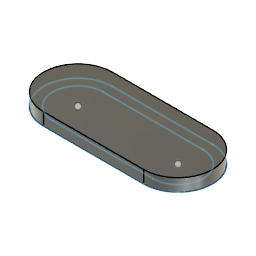
CNC (Autodesk Fusion 360 design; units mm, degrees)
part number: 2025-10-28-20-52-08-507
Autodesk Fusion 360 part; units mm, degrees
sketch "Sketch1" plane through (0, 0, 0) normal (0, 0, 1) x (1, 0, 0)
  line L0 (0.0245, 49.9718) -> (160.0245, 49.9718)
  line L1 (0.0257, -60.0282) -> (160.0257, -60.0282)
  arc A0 (0.0245, 49.9718) -> (0.0257, -60.0282) centre (-0.0009, -5.0282) ccw
  arc A1 (160.0257, -60.0282) -> (160.0245, 49.9718) centre (160.0195, -5.0282) ccw
  line L2 (80.0245, 49.9718) -> (80.0245, 34.9718) construction
  line L3 (0.0245, 34.9718) -> (160.0245, 34.9718)
  line L4 (80.0257, -60.0282) -> (80.0257, -45.0282) construction
  line L5 (0.0257, -45.0282) -> (160.0257, -45.0282)
  line L6 (160.0245, 49.9718) -> (160.0245, 34.9718) construction
  line L7 (160.0257, -60.0282) -> (160.0257, -45.0282) construction
  arc A2 (0.0245, 34.9718) -> (0.0257, -45.0282) centre (-0.0009, -5.0282) ccw
  arc A3 (160.0141, -45.0282) -> (160.0152, 34.9718) centre (160.0195, -5.0282) ccw
  dimension "d3" = 160
  dimension "d5" = 110
  dimension "d6" = 160
  dimension "d7" = 110
  dimension "d8" = 15
  dimension "d9" = 160
  dimension "d10" = 15
  dimension "d11" = 160
  dimension "d12" = 15
  dimension "d13" = 15
  dimension "d14" = 80
  dimension "d15" = 80
  constraint horizontal L0
  constraint horizontal L1
  constraint midpoint L0 L2.start
  constraint perpendicular L0 L2
  constraint horizontal L3
  constraint coincident L2.end L3
  constraint midpoint L1 L4.start
  constraint perpendicular L1 L4
  constraint horizontal L5
  constraint coincident L4.end L5
  constraint perpendicular L0 L6
  constraint coincident L3.end L6.end
  constraint perpendicular L1 L7
  constraint coincident L5.end L7.end
  constraint concentric A0 A2
  constraint concentric A1 A3
  constraint tangent L3 A2
  constraint tangent L3 A3
  constraint tangent L5 A2
  constraint tangent L5 A3
  constraint coincident L3 A3.end
  constraint coincident L5 A3.start
  measures "d3" distance of L0.start L0.end
  measures "d5" diameter of A0
  measures "d6" distance of L1.start L1.end
  measures "d7" diameter of A1
  measures "d8" distance of L2.start L2.end
  measures "d9" distance of L3.start L3.end
  measures "d10" distance of L4.start L4.end
  measures "d11" distance of L5.start L5.end
  measures "d12" distance of L0.end L3.end
  measures "d13" distance of L1.end L5.end
  measures "d14" diameter of A2
  measures "d15" diameter of A3
extrude "Extrude1" add sketch "Sketch1" along normal blind 20 contours L0 L1 A0 A1 | L3 L5 A2 A3
extrude "Extrude2" cut sketch "Sketch1" along normal blind 15 contours L3 L5 A2 A3
equation "length = 160 mm"
equation "width = 110 mm"
equation "d3 = length"
equation "thickness = 15 mm"
equation "d5 = width"
equation "d6 = length"
equation "d7 = width"
equation "d8 = thickness"
equation "d9 = length"
equation "d10 = thickness"
equation "d11 = length"
equation "d12 = thickness"
equation "d13 = thickness"
equation "d14 = width - thickness * 2"
equation "d15 = width - thickness * 2"
equation "o_extrude = 20 mm"
equation "i_extrude = 15 mm"
equation "d18 = o_extrude"
equation "d20 = i_extrude"
